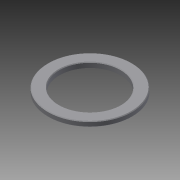
# Autodesk Inventor part: ThrustBearing-UpperRing
Saved by Autodesk Inventor 2015 (Build 190159000, 159)
## iProperties
Created: 2014-04-13
Part Number: ThrustBearing-UpperRing
Material: Generic
Document SubType Name: Modeling
Designer: Will Stuckey
Density: 1 g/cm^3
Appearance: Default
Author: Will Stuckey
Autodesk Inventor part; units mm, degrees
ref_plane "YZ Plane" through (0, 0, 0) normal (1, 0, 0) x (0, 1, 0)
ref_plane "XZ Plane" through (0, 0, 0) normal (0, 1, 0) x (-1, 0, 0)
ref_plane "XY Plane" through (0, 0, 0) normal (0, 0, 1) x (1, 0, 0)
sketch "Sketch1" plane through (0, 0, 0) normal (0, 1, 0) x (-1, 0, 0)
  circle A0 centre (0, 0) radius 26.1938
  circle A1 centre (0, 0) radius 19.05
  dimension "d0" = 52.3875
  dimension "d1" = 38.1
  constraints: 2 centre point, 2 coincident
  measures "d0" diameter of A0
  measures "d1" diameter of A1
extrude "Extrusion1" add sketch "Sketch1" along normal blind 3.175
sketch "Sketch2" plane through (0, 0, 0) normal (0, 0, 1) x (1, 0, 0)
  line L0 (-21.8281, 0) -> (-21.8281, -1.5875)
  circle A0 centre (-21.8281, -1.5875) radius 2.7781
  line L1 (0, 0) -> (0, 3.175)
  line L2 (26.1938, 3.175) -> (-26.1938, 3.175) projected
  dimension "d4" = 1.5875
  dimension "d5" = 5.5563
  constraints: 4 end point, 1 centre point, 1 coincident, 1 midpoint, 1 vertical
  measures "d4" distance of L0.start L0.end
  measures "d5" diameter of A0
revolve "Revolution1" cut sketch "Sketch2" angle 360 about axis through (0, 0, 0) along (0, 1, 0)
chamfer "Chamfer1" distance 0.3969 angle 45 1 edges at (26.1938, 3.175, 0)
chamfer "Chamfer2" distance 0.3969 angle 45 1 edges at (26.1938, 0, 0)
chamfer "Chamfer3" distance 0.3969 angle 45 1 edges at (19.05, 3.175, 0)
body "Solid1"
